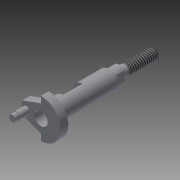
# Autodesk Inventor part: CrankShaft
Saved by Autodesk Inventor 2015 (Build 190159000, 159)
## iProperties
Created: 2016-02-13
Part Number: CrankShaft
Material: Generic
Document SubType Name: Modeling
Designer: Owner
Density: 1 g/cm^3
Appearance: Default
Mass: 2.43323 g
Surface Area: 23.2603 cm^2
Volume: 2.43323 cm^3
Author: Owner
Autodesk Inventor part; units mm, degrees
ref_plane "YZ Plane" through (0, 0, 0) normal (1, 0, 0) x (0, 1, 0)
ref_plane "XZ Plane" through (0, 0, 0) normal (0, 1, 0) x (-1, 0, 0)
ref_plane "XY Plane" through (0, 0, 0) normal (0, 0, 1) x (1, 0, 0)
sketch "Sketch1" plane through (0, 0, 0) normal (0, 0, 1) x (1, 0, 0)
  circle A0 centre (0, 0) radius 9.4742
  dimension "d0" = 18.9484
  constraints: 1 centre point, 1 coincident
  measures "d0" diameter of A0
extrude "Extrusion1" add sketch "Sketch1" against normal blind 3.81
sketch "Sketch2" plane through (0, 0, 0) normal (0, 0, 1) x (1, 0, 0)
  circle A0 centre (0, 0) radius 4.5085
  dimension "d3" = 9.017
  constraints: 1 centre point, 1 coincident
  measures "d3" diameter of A0
extrude "Extrusion2" add sketch "Sketch2" against normal blind 32.639
sketch "Sketch3" plane through (0, 0, 0) normal (0, 0, 1) x (1, 0, 0)
  circle A0 centre (0, 0) radius 3.4925
  dimension "d6" = 6.985
  constraints: 1 centre point, 1 coincident
  measures "d6" diameter of A0
extrude "Extrusion3" add sketch "Sketch3" against normal blind 38.1
sketch "Sketch4" plane through (0, 0, 0) normal (0, 0, 1) x (1, 0, 0)
  circle A0 centre (0, 0) radius 2.413
  dimension "d9" = 4.826
  constraints: 1 centre point, 1 coincident
  measures "d9" diameter of A0
extrude "Extrusion4" add sketch "Sketch4" against normal blind 54.61
sketch "Sketch6" plane through (0, 0, 0) normal (0, 0, 1) x (1, 0, 0)
  circle A0 centre (0, 0) radius 9.4742 projected
hole "Hole1" at (0, 0, 0) direction (0, 0, -1) diameter 6.5278 depth 22.352
sketch "Sketch5" plane through (0, 0, 0) normal (0, 1, 0) x (-1, 0, 0)
  line L0 (-4.5085, -32.639) -> (4.5085, -32.639) projected
  line L1 (4.5085, -3.81) -> (-4.5085, -3.81) projected
  line L2 (-3.4925, -38.1) -> (3.4925, -38.1) projected
  line L3 (3.4925, -32.639) -> (-3.4925, -32.639) projected
  line L4 (-3.4925, -32.639) -> (-3.4925, -38.1) projected
  line L5 (-2.413, -38.1) -> (-2.413, -54.61) projected
  line L6 (3.4925, -32.639) -> (3.4925, -38.1) projected
  line L7 (4.5085, -3.81) -> (4.5085, -32.639) projected
  line L8 (-4.5085, -3.81) -> (-4.5085, -32.639) projected
  line L9 (9.4742, 0) -> (9.4742, -3.81) projected
  line L10 (-9.4742, -3.81) -> (9.4742, -3.81) projected
  line L11 (-9.4742, 0) -> (9.4742, 0) projected
  line L12 (-9.4742, 0) -> (-9.4742, -3.81) projected
  line L13 (2.413, -38.1) -> (2.413, -54.61) projected
  line L14 (-2.413, -54.61) -> (2.413, -54.61) projected
  line L15 (-3.4925, -32.639) -> (-3.4925, -34.036) construction
  line L16 (-3.4925, -38.1) -> (3.4925, -38.1) projected
  line L17 (-3.4925, -34.036) -> (-2.5273, -34.036)
  line L18 (-2.5273, -34.036) -> (-2.5273, -38.1)
  line L19 (-2.5273, -38.1) -> (-3.4925, -38.1)
  line L20 (-3.4925, -38.1) -> (-3.4925, -34.036)
  line L21 (3.4925, -34.036) -> (2.5273, -34.036)
  line L22 (2.5273, -34.036) -> (2.5273, -38.1)
  line L23 (2.5273, -38.1) -> (3.4925, -38.1)
  line L24 (3.4925, -38.1) -> (3.4925, -34.036)
  point P0 (0, 0)
  dimension "d12" = 1.397
  dimension "d13" = 0.9652
  dimension "d14" = 0.9652
  constraints: 18 end point, 4 parallel, 4 point on line, 2 horizontal, 2 perpendicular
  measures "d12" distance of L4.start L15.end
  measures "d13" distance of L18.end L19.end
  measures "d14" distance of L23.end L22.end
extrude "Extrusion5" cut sketch "Sketch5" along normal through all both and the other way through all contours L17 L18 L2 L4 | L6 L2 L22 L21
sketch "Sketch7" plane through (0, 0, 0) normal (0, 1, 0) x (-1, 0, 0)
  line L0 (-9.4742, 0) -> (9.4742, 0) projected
  line L1 (9.4742, 0) -> (9.4742, -3.81) projected
  line L2 (4.5085, -3.81) -> (4.5085, -32.639) projected
  line L3 (3.2639, -22.352) -> (3.2639, 0) projected
  line L4 (-3.2639, -22.352) -> (-3.2639, 0) projected
  line L5 (3.2639, -22.352) -> (-3.2639, -22.352) projected
  line L6 (-4.5085, -3.81) -> (-4.5085, -32.639) projected
  line L7 (-9.4742, 0) -> (-9.4742, -3.81) projected
  line L8 (3.4925, -32.639) -> (3.4925, -34.036) projected
  line L9 (3.4925, -34.036) -> (2.5273, -34.036) projected
  line L10 (2.5273, -38.1) -> (2.5273, -34.036) projected
  line L11 (2.413, -38.1) -> (2.413, -54.61) projected
  line L12 (-2.413, -38.1) -> (-2.413, -54.61) projected
  line L13 (-2.5273, -34.036) -> (-2.5273, -38.1) projected
  line L14 (-3.4925, -32.639) -> (-3.4925, -34.036) projected
  line L15 (9.4742, 0) -> (9.4742, -10.668)
  line L16 (4.5085, -10.668) -> (-0.0127, -10.668)
  line L17 (-0.0127, -10.668) -> (-0.0127, -20.1168)
  line L18 (-0.0127, -20.1168) -> (4.5085, -20.1168)
  line L19 (4.5085, -20.1168) -> (4.5085, -10.668)
  point P0 (0, 0)
  dimension "d26" = 10.668
  dimension "d27" = 9.4488
  dimension "d42" = 4.5212
  constraints: 10 end point, 2 parallel, 1 horizontal, 1 perpendicular, 1 point on line, 1 vertical
  measures "d26" distance of L1.start L15.end
  measures "d27" distance of L17.end L16.end
  measures "d42" distance of L17.end L18.end
extrude "Extrusion6" cut sketch "Sketch7" along normal through all contours L16 L2 L18 L3 | L3 L18 L17 L16
sketch "Sketch9" plane through (0, 0, 0) normal (0, 0, 1) x (1, 0, 0)
  line L0 (0, 0) -> (-6.9342, 0)
  circle A0 centre (-6.9342, 0) radius 1.7399
  dimension "d35" = 6.9342
  dimension "d36" = 3.4798
  constraints: 2 end point, 1 centre point, 1 coincident, 1 horizontal
  measures "d35" distance of L0.start L0.end
  measures "d36" diameter of A0
extrude "Extrusion8" add sketch "Sketch9" along normal blind 4.826
sketch "Sketch10" plane through (-6.9342, 0, 4.826) normal (0, 0, 1) x (1, 0, 0)
  circle A0 centre (0, 0) radius 1.5875
  point P0 (6.9342, 0)
  dimension "d39" = 3.175
  constraints: 1 centre point
  measures "d39" diameter of A0
extrude "Extrusion9" add sketch "Sketch10" along normal blind 2.159
sketch "Sketch8" plane through (0, 0, 0) normal (0, 0, 1) x (1, 0, 0)
  circle A0 centre (0, 0) radius 9.4742 projected
  line L0 (0, -9.4742) -> (0, -6.2992)
  line L1 (0, -6.2992) -> (-8.9758, -3.0323)
  line L2 (0, 9.4742) -> (0, 6.2992)
  line L3 (0, 6.2992) -> (-8.9758, 3.0323)
  dimension "d30" = 3.175
  dimension "d31" = 110
  dimension "d32" = 3.175
  constraints: 8 end point, 4 point on circle, 2 vertical
  measures "d30" distance of L0.start L0.end
  measures "d31" angle of L1 L0
  measures "d32" distance of L2.start L2.end
extrude "Extrusion7" cut sketch "Sketch8" against normal through all contours L2 L3 A0 | A0 L1 L0
thread "Thread1" size "10-24 UNC" class "2A" standard "ANSI Unified Screw Threads" length 13.97
body "Solid1"
